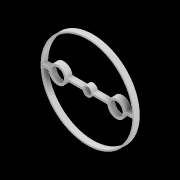
# Autodesk Inventor part: Magnet_rotor_parametriserad_02
Saved by Autodesk Inventor 2020 (Build 240168000, 168)
## iProperties
Created: 2020-11-21
Part Number: Magnet_rotor_parametriserad_02
Material: Generic
Document SubType Name: Modeling
Designer: Gottfrid
Density: 1 g/cm^3
Appearance: Default
D_inreRing_i: 6,500 mm
d_inreRing: 2,000 mm
d_toleransRing: 0,400 mm
r_filletAxel: 0,500 mm
Author: Gottfrid
Autodesk Inventor part; units mm, degrees
ref_plane "YZ Plane" through (0, 0, 0) normal (1, 0, 0) x (0, 1, 0)
ref_plane "XZ Plane" through (0, 0, 0) normal (0, 1, 0) x (-1, 0, 0)
ref_plane "XY Plane" through (0, 0, 0) normal (0, 0, 1) x (1, 0, 0)
sketch "Sketch1" plane through (0, 0, 0) normal (0, 0, 1) x (1, 0, 0)
  circle A0 centre (0, 0) radius 40
  circle A1 centre (0, 0) radius 41.25
  circle A2 centre (0, 0) radius 3.25
  circle A3 centre (0, 0) radius 4.25
  circle A4 centre (26, 0) radius 6.7
  circle A5 centre (26, 0) radius 7.7
  line L0 (0, 0) -> (43.8957, 0) construction
  line L1 (4.1536, 0.9) -> (18.3528, 0.9)
  line L2 (33.6472, 0.9) -> (39.9899, 0.9)
  line L3 (4.1536, -0.9) -> (18.3528, -0.9)
  line L4 (33.6472, -0.9) -> (39.9899, -0.9)
  line L5 (-4.1536, -0.9) -> (-18.3528, -0.9)
  line L6 (-4.1536, 0.9) -> (-18.3528, 0.9)
  circle A6 centre (-26, 0) radius 7.7
  circle A7 centre (-26, 0) radius 6.7
  line L7 (-33.6472, 0.9) -> (-39.9899, 0.9)
  line L8 (-33.6472, -0.9) -> (-39.9899, -0.9)
  line L9 (1.1569, -3.5962) -> (-1.1569, -3.5962)
  line L10 (-1.6569, -3.0962) -> (-1.6569, 3.0962)
  line L11 (-1.1569, 3.5962) -> (1.1569, 3.5962)
  line L12 (1.6569, 3.0962) -> (1.6569, -3.0962)
  line L13 (1.6569, -3.5962) -> (-1.6569, 3.5962) construction
  line L14 (-1.6569, -3.5962) -> (1.6569, 3.5962) construction
  arc A8 (-1.1569, 3.5962) -> (-1.6569, 3.0962) centre (-1.1569, 3.0962) ccw
  arc A9 (1.6569, 3.0962) -> (1.1569, 3.5962) centre (1.1569, 3.0962) ccw
  arc A10 (1.1569, -3.5962) -> (1.6569, -3.0962) centre (1.1569, -3.0962) ccw
  arc A11 (-1.6569, -3.0962) -> (-1.1569, -3.5962) centre (-1.1569, -3.0962) ccw
  point P0 (-1.6569, -2.7959)
  point P1 (-1.6569, 2.7959)
  point P2 (1.6569, 2.7959)
  point P3 (1.6569, -2.7959)
  dimension "d0" = 80
  dimension "d3" = 8.5
  dimension "d1" = 82.5
  dimension "d2" = 6.5
  dimension "d4" = 13.4
  dimension "d5" = 26
  dimension "d6" = 15.4
  dimension "d10" = 0.9
  dimension "d11" = 0.9
  dimension "d14" = 360
  dimension "d16" = 7.1923
  dimension "d17" = 3.3137
  dimension "d18" = 0.5
  constraints: 30 end point, 12 point on circle, 10 centre point, 8 coincident, 8 point on line, 8 tangent, 4 horizontal, 4 symmetric about line, 3 equal radius, 2 midpoint, 2 parallel, 1 horizontal alignment, 1 perpendicular, 39 other
  measures "d1" diameter of A1
  measures "d2" diameter of A2
  measures "d4" diameter of A4
  measures "d5" distance of A4.centre point (0, 0)
  measures "d6" diameter of A5
  measures "d10" vertical distance of L1.start point (0, 0)
  measures "d11" distance between parallel lines of L0 L2
  measures "d16" distance between parallel lines of L9 L11
  measures "d17" distance between parallel lines of L12 L10
  measures "d18" radius of A8
extrude "Extrusion1" add sketch "Sketch1" along normal blind 5 contours A0 L4 A5 L2 | L7 A6 L8 A0 | A5 | A6 | A5 L3 A3 L1 | L6 A3 L5 A6 | A3 | A1
sketch "Sketch2" plane through (0, 0, 5) normal (0, 0, 1) x (1, 0, 0)
  arc A0 (33.6472, 0.9) -> (18.3528, 0.9) centre (26, 0) ccw projected
  circle A1 centre (26, 0) radius 7.7
  circle A2 centre (26, 0) radius 5.8
  arc A3 (18.3528, -0.9) -> (33.6472, -0.9) centre (26, 0) ccw projected
  circle A4 centre (-26, 0) radius 5.8
  circle A5 centre (-26, 0) radius 7.7
  point P0 (0, 0)
  point P1 (18.3528, 0.9)
  point P2 (33.6472, 0.9)
  point P3 (-18.3528, 0.9)
  point P4 (-33.6472, 0.9)
  dimension "d21" = 7.7
  dimension "d22" = 11.6
  dimension "d27" = 360
  constraints: 4 centre point, 2 coincident, 1 concentric, 13 other
  measures "d21" radius of A0
  measures "d22" diameter of A2
extrude "Extrusion2" add sketch "Sketch2" along normal blind 0.4
equation "\"d0\" = D_yttreRing_i"
equation "\"d3\" = D_inreRing_i + d_inreRing"
equation "\"d1\" = D_yttreRing_i + d_yttreRing"
equation "\"d2\" = D_inreRing_i"
equation "\"d4\" = D_magnet + d_toleransRing"
equation "\"d5\" = l_magnetHållarRingFrånOrigo"
equation "\"d6\" = d_toleransRing + D_magnet + d_magnetHållarRing"
equation "\"d10\" = 0.5 * d_stöttor"
equation "\"d11\" = 0.5 * d_stöttor"
equation "\"d18\" = r_filletAxel"
equation "\"d19\" = h_höjdMagnetRotor"
equation "\"d22\" = D_magnet - d_magnetSkydd"
equation "\"d23\" = h_magnetSkydd"
equation "\"D_yttreRing_i\" = 80"
equation "\"d_yttreRing\" = 2.5"
equation "\"D_magnet\" = 13"
equation "\"D_inreRing_i\" = 6.5"
equation "\"d_inreRing\" = 2"
equation "\"h_höjdMagnetRotor\" = 5"
equation "\"d_stöttor\" = 1.8"
equation "\"d_toleransRing\" = 0.4"
equation "\"d_magnetHållarRing\" = 2"
equation "\"l_magnetHållarRingFrånOrigo\" = 26"
equation "\"r_filletAxel\" = 0.5"
equation "\"h_magnetSkydd\" = 0.4"
equation "\"d_magnetSkydd\" = 1.4"
body "Solid1"
